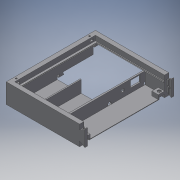
# Autodesk Inventor part: Case_side_back
Saved by Autodesk Inventor 2016 SP2 (Build 200236200, 236)
## iProperties
Created: 2018-06-26
Part Number: Case_side_back
Material: Generisch
Document SubType Name: Modeling
Designer: Nils
Density: 1 g/cm^3
Appearance: Vorgabe
Author: Nils
Autodesk Inventor part; units mm, degrees
ref_plane "YZ Plane" through (0, 0, 0) normal (1, 0, 0) x (0, 1, 0)
ref_plane "XZ Plane" through (0, 0, 0) normal (0, 1, 0) x (-1, 0, 0)
ref_plane "XY Plane" through (0, 0, 0) normal (0, 0, 1) x (1, 0, 0)
sketch "Skizze1" plane through (0, 0, 0) normal (0, 0, 1) x (1, 0, 0)
  circle A0 centre (1833.4019, 234.6963) radius 1.5 construction
  circle A1 centre (1833.4019, 396.1963) radius 1.5 construction
  line L0 (1838.4019, 230.6963) -> (1689.0019, 230.6963) construction
  line L1 (1689.0019, 230.6963) -> (1689.0019, 400.1963) construction
  line L2 (1689.0019, 400.1963) -> (1838.4019, 400.1963) construction
  line L3 (1838.4019, 400.1963) -> (1838.4019, 392.1963) construction
  line L4 (1838.4019, 392.1963) -> (1697.0019, 392.1963) construction
  line L5 (1697.0019, 392.1963) -> (1697.0019, 238.6963) construction
  line L6 (1697.0019, 238.6963) -> (1838.4019, 238.6963) construction
  line L7 (1838.4019, 238.6963) -> (1838.4019, 230.6963) construction
  line L8 (1828.4019, 390.6963) -> (1828.4019, 400.1963) construction
  line L9 (1828.4019, 230.6963) -> (1828.4019, 240.1963) construction
  line L10 (1828.4019, 230.6963) -> (1828.4019, 238.6963)
  line L11 (1828.4019, 238.6963) -> (1697.0019, 238.6963)
  line L12 (1697.0019, 238.6963) -> (1697.0019, 392.1963)
  line L13 (1828.4019, 392.1963) -> (1697.0019, 392.1963)
  line L14 (1828.4019, 392.1963) -> (1828.4019, 400.1963)
  line L15 (1828.4019, 400.1963) -> (1689.0019, 400.1963)
  line L16 (1689.0019, 400.1963) -> (1689.0019, 230.6963)
  line L17 (1689.0019, 230.6963) -> (1828.4019, 230.6963)
  circle A2 centre (1693.0019, 245.6963) radius 1.5 projected
  circle A3 centre (1693.0019, 385.1963) radius 1.5 projected
  point P0 (0, 0)
  constraints: 16 end point, 6 collinear, 4 point on line, 1 parallel
extrude "Extrusion1" add sketch "Skizze1" along normal blind 9.3 contours L17 L16 L15 L14 L13 L12 L11 L10 | A2 | A3
sketch "Skizze2" plane through (0, 0, 0) normal (0, 0, -1) x (-1, 0, 0)
  circle A0 centre (-1693.0019, 245.6963) radius 3 projected
  circle A1 centre (-1693.0019, 385.1963) radius 3 projected
  line L0 (-1689.0019, 400.1963) -> (-1689.0019, 230.6963) projected
  line L1 (-1689.0019, 230.6963) -> (-1828.4019, 230.6963) projected
  line L2 (-1828.4019, 230.6963) -> (-1828.4019, 240.1963) projected
  line L3 (-1828.4019, 240.1963) -> (-1701.0019, 240.1963) projected
  line L4 (-1701.0019, 240.1963) -> (-1701.0019, 390.6963) projected
  line L5 (-1701.0019, 390.6963) -> (-1828.4019, 390.6963) projected
  line L6 (-1828.4019, 390.6963) -> (-1828.4019, 400.1963) projected
  line L7 (-1828.4019, 400.1963) -> (-1689.0019, 400.1963) projected
  point P0 (0, 0)
extrude "Extrusion2" add sketch "Skizze2" along normal blind 2 contours A0 | A1 | L0 L1 L2 L3 L4 L5 L6 L7
chamfer "Fase1" distance 1.5 angle 45 3 edges at (1764.7019, 390.6963, -2) (1701.0019, 315.4463, -2) (1764.7019, 240.1963, -2)
sketch "Skizze3" plane through (0, 0, -2) normal (0, 0, -1) x (-1, 0, 0)
  line L0 (-1699.5019, 392.1963) -> (-1828.4019, 392.1963) projected
  line L1 (-1699.5019, 238.6963) -> (-1699.5019, 392.1963) projected
  line L2 (-1828.4019, 238.6963) -> (-1699.5019, 238.6963) projected
  line L3 (-1828.4019, 238.6963) -> (-1828.4019, 230.6963) projected
  line L4 (-1828.4019, 230.6963) -> (-1689.0019, 230.6963) projected
  line L5 (-1689.0019, 230.6963) -> (-1689.0019, 400.1963) projected
  line L6 (-1689.0019, 400.1963) -> (-1828.4019, 400.1963) projected
  line L7 (-1828.4019, 400.1963) -> (-1828.4019, 392.1963) projected
  point P0 (0, 0)
extrude "Extrusion3" add sketch "Skizze3" along normal blind 26
sketch "Skizze4" plane through (0, 0, -28) normal (0, 0, -1) x (-1, 0, 0)
  line L0 (-1828.4019, 392.1963) -> (-1828.4019, 400.1963) projected
  line L1 (-1828.4019, 392.1963) -> (-1699.5019, 392.1963)
  line L2 (-1699.5019, 392.1963) -> (-1699.5019, 238.6963)
  line L3 (-1699.5019, 238.6963) -> (-1828.4019, 238.6963)
  line L4 (-1828.4019, 238.6963) -> (-1828.4019, 392.1963)
  line L5 (-1699.5019, 392.1963) -> (-1699.5019, 238.6963) projected
  line L6 (-1699.5019, 238.6963) -> (-1828.4019, 238.6963) projected
  point P0 (0, 0)
  constraints: 8 end point, 2 collinear, 2 parallel, 1 horizontal, 1 perpendicular
extrude "Extrusion4" add sketch "Skizze4" against normal blind 3
sketch "Skizze6" plane through (0, 0, -25) normal (0, 0, 1) x (1, 0, 0)
  line L0 (1828.4019, 238.6963) -> (1697.0019, 238.6963) projected
  line L1 (1743.0019, 238.6963) -> (1745.0019, 238.6963)
  line L2 (1745.0019, 238.6963) -> (1745.0019, 317.1963)
  line L3 (1745.0019, 317.1963) -> (1743.0019, 317.1963)
  line L4 (1743.0019, 317.1963) -> (1743.0019, 238.6963)
  line L5 (1697.0019, 238.6963) -> (1697.0019, 392.1963) projected
  line L6 (1791.5019, 238.6963) -> (1791.5019, 392.1963)
  line L7 (1791.5019, 392.1963) -> (1789.0019, 392.1963)
  line L8 (1697.0019, 392.1963) -> (1828.4019, 392.1963) projected
  line L9 (1789.0019, 392.1963) -> (1789.0019, 317.1963)
  line L10 (1789.0019, 317.1963) -> (1788.5019, 317.1963)
  line L11 (1788.5019, 317.1963) -> (1788.5019, 238.6963)
  line L12 (1791.5019, 238.6963) -> (1788.5019, 238.6963)
  line L13 (1789.0019, 390.6963) -> (1789.0019, 392.1963)
  line L14 (1789.0019, 392.1963) -> (1791.5019, 392.1963)
  line L15 (1791.5019, 392.1963) -> (1791.5019, 390.6963)
  point P0 (0, 0)
  point P1 (1699.5019, 238.6963)
  dimension "d15" = 2
  dimension "d16" = 78.5
  dimension "d18" = 2.5
  dimension "d20" = 90
  dimension "d21" = 43.5
  dimension "d22" = 3
  dimension "d23" = 0.5
  dimension "d24" = 78.5
  dimension "d150" = 43.5
  constraints: 26 end point, 6 point on line, 5 perpendicular, 2 collinear, 2 parallel, 1 horizontal
  measures "d15" distance of L3.end L2.end
  measures "d16" distance of L2.end L1.end
  measures "d18" distance of L6.end L7.end
  measures "d20" angle of L9 L10
  measures "d21" distance between parallel lines of L2 L11
  measures "d22" distance between parallel lines of L11 L6
  measures "d23" distance of L9.end L10.end
  measures "d24" distance of L10.end L11.end
  measures "d150" distance of L1.start point (1699.502, 238.696)
extrude "Extrusion5" add sketch "Skizze6" along normal blind 23 contours L0 L11 L10 L9 L7 L6 | L0 L4 L3 L2
sketch "Skizze9" plane through (0, 0, -25) normal (0, 0, 1) x (1, 0, 0)
  line L0 (1828.4019, 230.6963) -> (1828.4019, 238.6963) projected
  line L1 (1828.4019, 238.6963) -> (1816.4019, 238.6963)
  line L2 (1816.4019, 238.6963) -> (1816.4019, 250.6963)
  line L3 (1816.4019, 250.6963) -> (1828.4019, 250.6963)
  line L4 (1828.4019, 250.6963) -> (1828.4019, 238.6963)
  line L5 (1828.4019, 392.1963) -> (1828.4019, 400.1963) projected
  line L6 (1828.4019, 392.1963) -> (1816.4019, 392.1963)
  line L7 (1816.4019, 392.1963) -> (1816.4019, 380.1963)
  line L8 (1816.4019, 380.1963) -> (1828.4019, 380.1963)
  line L9 (1828.4019, 380.1963) -> (1828.4019, 392.1963)
  point P0 (0, 0)
  dimension "d41" = 12
  dimension "d42" = 12
  dimension "d43" = 12
  dimension "d44" = 12
  constraints: 16 end point, 4 parallel, 2 horizontal, 2 perpendicular
  measures "d41" distance of L2.end L3.end
  measures "d42" distance of L1.end L2.end
  measures "d43" distance of L8.end L7.end
  measures "d44" distance of L7.end L6.end
extrude "Extrusion8" add sketch "Skizze9" along normal blind 8
sketch "Skizze10" plane through (0, 0, -28) normal (0, 0, -1) x (-1, 0, 0)
  line L0 (-1828.4019, 238.6963) -> (-1816.4019, 238.6963) projected
  line L1 (-1816.4019, 392.1963) -> (-1828.4019, 392.1963) projected
  line L2 (-1828.4019, 392.1963) -> (-1828.4019, 390.6963) projected
  line L3 (-1697.0019, 238.6963) -> (-1828.4019, 238.6963) projected
  line L4 (-1828.4019, 392.1963) -> (-1818.4019, 392.1963)
  line L5 (-1818.4019, 392.1963) -> (-1818.4019, 238.6963)
  line L6 (-1818.4019, 238.6963) -> (-1828.4019, 238.6963)
  line L7 (-1828.4019, 238.6963) -> (-1828.4019, 392.1963)
  point P0 (0, 0)
  dimension "d47" = 10
  constraints: 8 end point, 2 parallel, 1 horizontal, 1 perpendicular, 1 point on line
  measures "d47" distance of L5.end L6.end
extrude "Extrusion9" cut sketch "Skizze10" against normal blind 2
sketch "Skizze11" plane through (0, 0, -26) normal (0, 0, -1) x (-1, 0, 0)
  line L0 (-1828.4019, 238.6963) -> (-1828.4019, 230.6963) projected
  line L1 (-1828.4019, 238.6963) -> (-1818.4019, 238.6963)
  line L2 (-1818.4019, 238.6963) -> (-1818.4019, 248.6963)
  line L3 (-1818.4019, 248.6963) -> (-1828.4019, 248.6963)
  line L4 (-1828.4019, 248.6963) -> (-1828.4019, 238.6963)
  line L5 (-1828.4019, 392.1963) -> (-1818.4019, 392.1963) projected
  line L6 (-1828.4019, 392.1963) -> (-1818.4019, 392.1963)
  line L7 (-1818.4019, 392.1963) -> (-1818.4019, 382.1963)
  line L8 (-1818.4019, 382.1963) -> (-1828.4019, 382.1963)
  line L9 (-1828.4019, 382.1963) -> (-1828.4019, 392.1963)
  point P0 (0, 0)
  dimension "d50" = 10
  dimension "d51" = 10
  dimension "d52" = 10
  dimension "d53" = 10
  constraints: 16 end point, 4 parallel, 2 horizontal, 2 perpendicular
  measures "d50" distance of L3.end L2.end
  measures "d51" distance of L2.end L1.end
  measures "d52" distance of L7.end L8.end
  measures "d53" distance of L6.end L7.end
extrude "Extrusion10" cut sketch "Skizze11" against normal blind 3.5
sketch "Skizze12" plane through (0, 0, -22.5) normal (0, 0, -1) x (-1, 0, 0)
  line L0 (-1818.4019, 238.6963) -> (-1828.4019, 238.6963) construction
  line L1 (-1818.4019, 248.6963) -> (-1818.4019, 238.6963) construction
  line L2 (-1828.4019, 248.6963) -> (-1818.4019, 248.6963) construction
  line L3 (-1828.4019, 238.6963) -> (-1828.4019, 248.6963) construction
  line L4 (-1828.4019, 392.1963) -> (-1818.4019, 392.1963) construction
  line L5 (-1828.4019, 382.1963) -> (-1828.4019, 392.1963) construction
  line L6 (-1818.4019, 382.1963) -> (-1828.4019, 382.1963) construction
  line L7 (-1818.4019, 392.1963) -> (-1818.4019, 382.1963) construction
  circle A0 centre (-1823.4019, 243.6963) radius 1.5
  circle A1 centre (-1823.4019, 387.1963) radius 1.5
  line L8 (-1697.0019, 392.1963) -> (-1828.4019, 392.1963) construction
  line L9 (-1818.4019, 382.1963) -> (-1828.4019, 382.1963) construction
  line L10 (-1828.4019, 392.1963) -> (-1818.4019, 382.1963) construction
  line L11 (-1828.4019, 248.6963) -> (-1818.4019, 248.6963) construction
  line L12 (-1828.4019, 238.6963) -> (-1791.5019, 238.6963) construction
  line L13 (-1818.4019, 248.6963) -> (-1828.4019, 238.6963) construction
  point P0 (0, 0)
  dimension "d56" = 3
  dimension "d57" = 3
  constraints: 4 end point, 2 centre point, 2 midpoint
  measures "d56" diameter of A0
  measures "d57" diameter of A1
extrude "Extrusion11" cut sketch "Skizze12" against normal blind 9.25
sketch "Skizze13" plane through (0, 0, -17) normal (0, 0, 1) x (1, 0, 0)
  circle A0 centre (1823.4019, 243.6963) radius 1.5 projected
  circle A1 centre (1823.4019, 387.1963) radius 1.5 projected
  line L0 (1826.3019, 385.522) -> (1823.4019, 383.8476)
  line L1 (1823.4019, 383.8476) -> (1820.5019, 385.522)
  line L2 (1820.5019, 385.522) -> (1820.5019, 388.8706)
  line L3 (1820.5019, 388.8706) -> (1823.4019, 390.5449)
  line L4 (1823.4019, 390.5449) -> (1826.3019, 388.8706)
  line L5 (1826.3019, 388.8706) -> (1826.3019, 385.522)
  line L6 (1826.3019, 245.3706) -> (1826.3019, 242.022)
  line L7 (1826.3019, 242.022) -> (1823.4019, 240.3476)
  line L8 (1823.4019, 240.3476) -> (1820.5019, 242.022)
  line L9 (1820.5019, 242.022) -> (1820.5019, 245.3706)
  line L10 (1820.5019, 245.3706) -> (1823.4019, 247.0449)
  line L11 (1823.4019, 247.0449) -> (1826.3019, 245.3706)
  point P0 (0, 0)
  dimension "d64" = 5.8
  dimension "d65" = 5.8
  constraints: 24 end point, 2 coincident, 2 vertical, 26 other
  measures "d64" distance between parallel lines of L6 L9
  measures "d65" distance between parallel lines of L5 L2
extrude "Extrusion12" cut sketch "Skizze13" against normal blind 2.5
sketch "Skizze14" plane through (1689.0019, 230.6963, 9.3) normal (0, -1, 0) x (1, 0, 0)
  line L0 (139.4, 0) -> (139.4, -37.3) projected
  line L1 (139.4, -9.4235) -> (149.4, -3.65)
  line L2 (149.4, -3.65) -> (149.4, -33.65)
  line L3 (149.4, -33.65) -> (139.4, -27.8765)
  line L4 (139.4, -9.4235) -> (139.4, -27.8765)
  line L5 (139.4, 0) -> (149.4, -3.65) construction
  line L6 (149.4, -33.65) -> (139.4, -37.3) construction
  point P0 (-1689.0019, -9.3)
  dimension "d68" = 10
  dimension "d69" = 30
  dimension "d70" = 60
  dimension "d71" = 60
  constraints: 12 end point, 2 point on line, 1 collinear, 1 equal length, 1 parallel
  measures "d68" distance between parallel lines of L2 L0
  measures "d69" distance of L1.end L2.end
  measures "d70" angle of L1 L0
  measures "d71" angle of L0 L3
extrude "Extrusion13" add sketch "Skizze14" against normal blind 5
sketch "Skizze15" plane through (1689.0019, 400.1963, 9.3) normal (0, 1, 0) x (1, 0, 0)
  line L0 (139.4, 9.4235) -> (139.4, 27.8765) projected
  line L1 (139.4, 9.4235) -> (149.4, 3.65) projected
  line L2 (149.4, 3.65) -> (149.4, 33.65) projected
  line L3 (149.4, 33.65) -> (139.4, 27.8765) projected
  point P0 (-1689.0019, 9.3)
extrude "Extrusion14" add sketch "Skizze15" against normal blind 5
sketch "Skizze16" plane through (1789.0019, 317.1963, -28) normal (-1, 0, 0) x (0, 0, 1)
  line L0 (12, 30) -> (17, 30)
  line L1 (17, 30) -> (17, 35)
  line L2 (17, 35) -> (12, 35)
  line L3 (12, 35) -> (12, 30)
  line L4 (3, 0) -> (26, 0) projected
  line L5 (26, 75) -> (26, 0) projected
  point P0 (28, -317.1963)
  dimension "d76" = 5
  dimension "d77" = 5
  dimension "d217" = 30
  dimension "d218" = 9
  constraints: 8 end point, 2 parallel, 1 horizontal, 1 perpendicular
  measures "d76" distance of L2.end L1.end
  measures "d77" distance of L1.end L0.end
  measures "d217" distance between parallel lines of L4 L0
  measures "d218" distance between parallel lines of L5 L1
extrude "Extrusion15" cut sketch "Skizze16" against normal blind 2.5
sketch "Skizze17" plane through (1689.0019, 230.6963, 9.3) normal (-1, 0, 0) x (0, 0, 1)
  line L0 (-33.65, 0) -> (-3.65, 0) construction
  line L1 (-18.65, 0) -> (-18.65, 86.5) construction
  line L2 (-34.3, 86.5) -> (-11.3, 86.5) construction
  circle A0 centre (-18.65, 76.5) radius 5
  circle A1 centre (-18.65, 51.5) radius 5
  point P0 (-9.3, -230.6963)
  dimension "d82" = 10
  dimension "d83" = 10
  dimension "d84" = 25
  dimension "d85" = 10
  constraints: 3 point on line, 2 centre point, 2 end point, 1 midpoint, 1 vertical
  measures "d82" diameter of A0
  measures "d83" diameter of A1
  measures "d84" distance of A1.centre A0.centre
  measures "d85" distance from line of L2 A0.centre
extrude "Extrusion16" cut sketch "Skizze17" against normal blind 4
sketch "Skizze18" plane through (0, 0, 9.3) normal (0, 0, 1) x (1, 0, 0)
  circle A0 centre (1693.0019, 245.6963) radius 1.5 projected
  circle A1 centre (1693.0019, 385.1963) radius 1.5 projected
  point P0 (0, 0)
extrude "Extrusion17" cut sketch "Skizze18" against normal blind 9
sketch "Skizze19" plane through (1697.0019, 238.6963, 9.3) normal (1, 0, 0) x (0, 0, -1)
  line L0 (0, 8.5) -> (9, 8.5) construction
  line L1 (0, 5.5) -> (9, 5.5) construction
  line L2 (0, 148) -> (9, 148) construction
  line L3 (0, 145) -> (9, 145) construction
  line L4 (3.5, 143.65) -> (6.5, 143.65)
  line L5 (6.5, 143.65) -> (6.5, 149.35)
  line L6 (6.5, 149.35) -> (3.5, 149.35)
  line L7 (3.5, 149.35) -> (3.5, 143.65)
  line L8 (3.5, 9.85) -> (6.5, 9.85)
  line L9 (6.5, 9.85) -> (6.5, 4.15)
  line L10 (6.5, 4.15) -> (3.5, 4.15)
  line L11 (3.5, 4.15) -> (3.5, 9.85)
  line L12 (5, 4.15) -> (5, 5.5) construction
  line L13 (5, 8.5) -> (5, 9.85) construction
  line L14 (0, 0) -> (0, 153.5) construction
  point P0 (9.3, -238.6963)
  dimension "d90" = 3
  dimension "d91" = 5.7
  dimension "d92" = 3
  dimension "d93" = 5.7
  dimension "d94" = 1.35
  dimension "d95" = 3.5
  dimension "d98" = 1.35
  constraints: 20 end point, 4 parallel, 4 point on line, 3 perpendicular, 2 horizontal, 2 midpoint, 1 collinear
  measures "d90" distance of L6.end L5.end
  measures "d91" distance of L5.end L4.end
  measures "d92" distance of L9.end L10.end
  measures "d93" distance of L8.end L9.end
  measures "d94" distance between parallel lines of L6 L2
  measures "d95" distance between parallel lines of L7 L14
  measures "d98" distance between parallel lines of L8 L0
extrude "Extrusion18" cut sketch "Skizze19" against normal blind 7
sketch "Skizze20" plane through (0, 0, 9.3) normal (0, 0, 1) x (1, 0, 0)
  circle A0 centre (1833.4019, 234.6963) radius 1.5 projected
  circle A1 centre (1833.4019, 396.1963) radius 1.5 projected
  point P0 (0, 0)
extrude "Extrusion19" cut sketch "Skizze20" against normal blind 62.25
sketch "Skizze21" plane through (1689.0019, 235.6963, 9.3) normal (0, 1, 0) x (1, 0, 0)
  line L0 (139.4, 9.4235) -> (139.4, 27.8765) construction
  line L1 (139.4, 18.65) -> (149.4, 18.65) construction
  line L2 (149.4, 3.65) -> (149.4, 33.65) construction
  line L3 (141.55, 17.25) -> (147.25, 17.25)
  line L4 (147.25, 17.25) -> (147.25, 20.05)
  line L5 (147.25, 20.05) -> (141.55, 20.05)
  line L6 (141.55, 20.05) -> (141.55, 17.25)
  line L7 (141.55, 17.25) -> (147.25, 20.05) construction
  line L8 (147.25, 17.25) -> (141.55, 20.05) construction
  point P0 (144.4, 18.65)
  dimension "d101" = 5.7
  dimension "d102" = 2.8
  constraints: 14 end point, 5 midpoint, 2 parallel, 1 horizontal, 1 perpendicular
  measures "d101" distance of L5.end L4.end
  measures "d102" distance of L4.end L3.end
extrude "Extrusion20" cut sketch "Skizze21" against normal blind 4
sketch "Skizze22" plane through (1689.0019, 395.1963, 9.3) normal (0, -1, 0) x (1, 0, 0)
  line L0 (147.25, -17.25) -> (141.55, -17.25) projected
  line L1 (147.25, -20.05) -> (147.25, -17.25) projected
  line L2 (141.55, -20.05) -> (147.25, -20.05) projected
  line L3 (141.55, -17.25) -> (141.55, -20.05) projected
  point P0 (-1689.0019, -9.3)
extrude "Extrusion21" cut sketch "Skizze22" against normal blind 4
sketch "Skizze27" plane through (1689.0019, 230.6963, 9.3) normal (-1, 0, 0) x (0, 0, 1)
  line L0 (-11.3, 161.5) -> (-11.3, 86.5) construction
  line L1 (-37.3, 161.5) -> (-37.3, 8) projected
  line L2 (-37.3, 86.5) -> (-27.3, 86.5)
  line L3 (-27.3, 86.5) -> (-27.3, 154.5)
  line L4 (-27.3, 154.5) -> (-11.3, 154.5)
  line L5 (-11.3, 154.5) -> (-11.3, 169.5)
  line L6 (-11.3, 169.5) -> (-37.3, 169.5)
  line L7 (-37.3, 169.5) -> (-37.3, 86.5)
  line L8 (0, 169.5) -> (-37.3, 169.5) projected
  line L9 (-34.3, 86.5) -> (-11.3, 86.5) construction
  point P0 (-9.3, -230.6963)
  dimension "d151" = 10
  dimension "d152" = 15
  constraints: 12 end point, 3 collinear, 3 perpendicular, 2 point on line, 1 vertical
  measures "d151" distance of L2.start L2.end
  measures "d152" distance between parallel lines of L6 L4
extrude "Extrusion22" cut sketch "Skizze27" against normal blind 100
sketch "Skizze28" plane through (1699.5019, 238.6963, -2) normal (1, 0, 0) x (0, 0, -1)
  line L0 (16, 78.5) -> (16, 146.5) projected
  line L1 (16, 82.8199) -> (21, 81)
  line L2 (21, 81) -> (21, 91)
  line L3 (21, 91) -> (16, 89.1801)
  line L4 (0, 146.5) -> (0, 153.5) projected
  line L5 (5, 159) -> (0, 157.1801)
  line L6 (0, 161.5) -> (0, 146.5) projected
  line L7 (0, 150.8199) -> (5, 149)
  line L8 (5, 149) -> (5, 159)
  line L9 (23, 78.5) -> (16, 78.5) projected
  point P0 (-2, -238.6963)
  dimension "d156" = 5
  dimension "d157" = 70
  dimension "d158" = 70
  dimension "d159" = 10
  dimension "d162" = 70
  dimension "d163" = 10
  dimension "d164" = 70
  dimension "d165" = 2.5
  dimension "d166" = 5
  dimension "d167" = 2.5
  constraints: 12 end point, 4 point on line, 2 parallel, 1 vertical
  measures "d156" distance between parallel lines of L0 L2
  measures "d157" angle of L3 L0
  measures "d158" angle of L0 L1
  measures "d159" distance of L1.end L2.end
  measures "d162" angle of L5 L6
  measures "d163" distance of L7.end L5.start
  measures "d164" angle of L7 L4
  measures "d165" vertical distance of L6.start L5.start
  measures "d166" distance between parallel lines of L8 L6
  measures "d167" distance from line of L1.end L9
extrude "Extrusion23" add sketch "Skizze28" against normal blind 6
sketch "Skizze29" plane through (1789.0019, 317.1963, -28) normal (-1, 0, 0) x (0, 0, 1)
  line L0 (5, 12.5) -> (5, 2.5) construction
  line L1 (5, 7.5) -> (5, 7.5) construction
  line L2 (21, 70.5) -> (21, 80.5) construction
  line L3 (21, 75.5) -> (0, 75.5) construction
  circle A0 centre (5, 75.5) radius 3.5
  circle A1 centre (5, 7.5) radius 3.5
  line L4 (0, 83) -> (26, 83) projected
  line L5 (0, 0) -> (0, 83) projected
  dimension "d170" = 7
  dimension "d171" = 7
  dimension "d172" = 7.5
  dimension "d173" = 5
  dimension "d174" = 5
  constraints: 4 end point, 3 midpoint, 2 centre point, 2 horizontal, 1 point on line
  measures "d170" diameter of A0
  measures "d171" diameter of A1
  measures "d172" distance from line of L4 A0.centre
  measures "d173" distance from line of L5 A0.centre
  measures "d174" distance from line of L5 A1.centre
extrude "Extrusion24" cut sketch "Skizze29" against normal blind 2.5
thread "Gewinde3" size "M10x1.5" class "6H" standard "ANSI Metric M Profile" full length
thread "Gewinde4" size "M10x1.5" class "6H" standard "ANSI Metric M Profile" full length
sketch "Skizze31" plane through (1693.0019, 307.1963, -9.35) normal (0, -1, 0) x (0, 0, 1)
  line L0 (5, 0) -> (5, 4)
  line L1 (5, 4) -> (4.0211, 4)
  line L2 (4.0211, 4) -> (4.0211, 0)
  line L3 (4.0211, 0) -> (5, 0)
  line L4 (0, -0.8) -> (0, 4.8) projected
  constraints: 8 end point
revolve "Umdrehung3" add sketch "Skizze31" angle 360 about axis through (1693.0019, 307.1963, -9.35) along (-1, 0, 0) separate body
sketch "Skizze30" plane through (1693.0019, 307.1963, -4.35) normal (0, 1, 0) x (-1, 0, 0)
  line L0 (-0.8887, -0.0802) -> (-0.7501, -0.0802) construction
  line L1 (0.1385, -0.899) -> (-0.0001, -1.1391) construction
  line L2 (-1.5001, -1.1391) -> (-1.6387, -0.899) construction
  line L3 (-0.6115, -0.0802) -> (-0.7501, 0.1599) construction
  line L4 (-0.7501, 0.1599) -> (-0.8887, -0.0802) construction
  line L5 (-1.5001, -1.1391) -> (-1.3615, -0.899) construction
  line L6 (-0.6115, -0.0802) -> (-0.1387, -0.899)
  line L7 (-1.6387, -0.899) -> (-1.3615, -0.899) construction
  arc A0 (-1.6387, -0.899) -> (-1.5001, -0.979) centre (-1.5001, -0.819) ccw construction
  line L8 (0.1385, -0.899) -> (-0.1387, -0.899) construction
  line L9 (-1.5001, -1.1391) -> (-1.5001, -0.899) construction
  line L10 (-0.0001, -1.1391) -> (-0.0001, -0.899) construction
  line L11 (-0.7501, 0.1599) -> (-0.7501, -0.0002) construction
  line L12 (-1.5001, -0.979) -> (-0.0001, -0.979)
  arc A1 (-1.5001, -0.979) -> (-1.3615, -0.899) centre (-1.5001, -0.819) ccw
  line L13 (-0.1387, -0.899) -> (-0.0001, -1.1391) construction
  line L14 (-1.3615, -0.899) -> (-0.8887, -0.0802)
  line L15 (-0.0001, -0.0002) -> (-0.0001, 0.0177)
  line L16 (-0.0001, 0.0177) -> (-0.0001, -0.0002)
  line L17 (-0.0001, -0.0002) -> (0.0334, -0.0002)
  arc A2 (-0.1387, -0.899) -> (-0.0001, -0.979) centre (-0.0001, -0.819) ccw
  arc A3 (-0.0001, -0.979) -> (0.1385, -0.899) centre (-0.0001, -0.819) ccw construction
  arc A4 (-0.7501, -0.0002) -> (-0.8887, -0.0802) centre (-0.7501, -0.1603) ccw
  arc A5 (-0.6115, -0.0802) -> (-0.7501, -0.0002) centre (-0.7501, -0.1603) ccw
  line L18 (-0.7501, -0.0002) -> (-0.7501, -0.0802) construction
  line L19 (-0.7501, -0.0802) -> (-0.6115, -0.0802) construction
  dimension "d181" = 60
  dimension "d182" = 0.2401
  dimension "d183" = 0.2401
  dimension "Skizze30_ThreadOffset" = 0
  dimension "Skizze30_MajorRadius" = 0.9789
  dimension "d186" = 1.5
  dimension "Skizze30_MinorRadius" = 0
  constraints: 40 end point, 12 point on circle, 10 parallel, 8 tangent, 6 centre point, 6 collinear, 2 midpoint, 2 point on line, 1 horizontal, 1 perpendicular, 3 other
  measures "d181" angle of L6 L14
  measures "d182" distance of L3.end L0.end
  measures "d183" distance of L1.end L10.end
  measures "Skizze30_ThreadOffset" distance between parallel lines of L15 L10
  measures "Skizze30_MajorRadius" distance from line of L12 L15.start
  measures "d186" distance from line of L1.end L9
  measures "Skizze30_MinorRadius" distance edge to line of A5 L17
coil "Spirale3" sketch "Skizze30" operation cut axis through (1693.0019, 307.1963, -9.35) along (-1, 0, 0) pitch 1.5015 turns 4.662005 hand right bodies 2
sketch "Skizze33" plane through (1693.0019, 282.1963, -9.35) normal (0, -1, 0) x (0, 0, 1)
  line L0 (5, 0) -> (5, 4)
  line L1 (5, 4) -> (4.0211, 4)
  line L2 (4.0211, 4) -> (4.0211, 0)
  line L3 (4.0211, 0) -> (5, 0)
  line L4 (0, -0.8) -> (0, 4.8) projected
  constraints: 8 end point
revolve "Umdrehung4" add sketch "Skizze33" angle 360 about axis through (1693.0019, 282.1963, -9.35) along (-1, 0, 0) separate body
sketch "Skizze32" plane through (1693.0019, 282.1963, -4.35) normal (0, 1, 0) x (-1, 0, 0)
  line L0 (-0.8887, -0.0802) -> (-0.7501, -0.0802) construction
  line L1 (0.1385, -0.899) -> (-0.0001, -1.1391) construction
  line L2 (-1.5001, -1.1391) -> (-1.6387, -0.899) construction
  line L3 (-0.6115, -0.0802) -> (-0.7501, 0.1599) construction
  line L4 (-0.7501, 0.1599) -> (-0.8887, -0.0802) construction
  line L5 (-1.5001, -1.1391) -> (-1.3615, -0.899) construction
  line L6 (-0.6115, -0.0802) -> (-0.1387, -0.899)
  line L7 (-1.6387, -0.899) -> (-1.3615, -0.899) construction
  arc A0 (-1.6387, -0.899) -> (-1.5001, -0.979) centre (-1.5001, -0.819) ccw construction
  line L8 (0.1385, -0.899) -> (-0.1387, -0.899) construction
  line L9 (-1.5001, -1.1391) -> (-1.5001, -0.899) construction
  line L10 (-0.0001, -1.1391) -> (-0.0001, -0.899) construction
  line L11 (-0.7501, 0.1599) -> (-0.7501, -0.0002) construction
  line L12 (-1.5001, -0.979) -> (-0.0001, -0.979)
  arc A1 (-1.5001, -0.979) -> (-1.3615, -0.899) centre (-1.5001, -0.819) ccw
  line L13 (-0.1387, -0.899) -> (-0.0001, -1.1391) construction
  line L14 (-1.3615, -0.899) -> (-0.8887, -0.0802)
  line L15 (-0.0001, -0.0002) -> (-0.0001, 0.0177)
  line L16 (-0.0001, 0.0177) -> (-0.0001, -0.0002)
  line L17 (-0.0001, -0.0002) -> (0.0334, -0.0002)
  arc A2 (-0.1387, -0.899) -> (-0.0001, -0.979) centre (-0.0001, -0.819) ccw
  arc A3 (-0.0001, -0.979) -> (0.1385, -0.899) centre (-0.0001, -0.819) ccw construction
  arc A4 (-0.7501, -0.0002) -> (-0.8887, -0.0802) centre (-0.7501, -0.1603) ccw
  arc A5 (-0.6115, -0.0802) -> (-0.7501, -0.0002) centre (-0.7501, -0.1603) ccw
  line L18 (-0.7501, -0.0002) -> (-0.7501, -0.0802) construction
  line L19 (-0.7501, -0.0802) -> (-0.6115, -0.0802) construction
  dimension "d199" = 60
  dimension "d200" = 0.2401
  dimension "d201" = 0.2401
  dimension "Skizze32_ThreadOffset" = 0
  dimension "Skizze32_MajorRadius" = 0.9789
  dimension "d204" = 1.5
  dimension "Skizze32_MinorRadius" = 0
  constraints: 40 end point, 12 point on circle, 10 parallel, 8 tangent, 6 centre point, 6 collinear, 2 midpoint, 2 point on line, 1 horizontal, 1 perpendicular, 3 other
  measures "d199" angle of L6 L14
  measures "d200" distance of L3.end L0.end
  measures "d201" distance of L1.end L10.end
  measures "Skizze32_ThreadOffset" distance between parallel lines of L15 L10
  measures "Skizze32_MajorRadius" distance from line of L12 L15.start
  measures "d204" distance from line of L1.end L9
  measures "Skizze32_MinorRadius" distance edge to line of A5 L17
coil "Spirale4" sketch "Skizze32" operation cut axis through (1693.0019, 282.1963, -9.35) along (-1, 0, 0) pitch 1.5015 turns 4.662005 hand right bodies 3
sketch "Skizze34" plane through (1789.0019, 317.1963, -28) normal (-1, 0, 0) x (0, 0, 1)
  line L0 (11.5, 47) -> (24, 47)
  line L1 (24, 47) -> (24, 66)
  line L2 (24, 66) -> (11.5, 66)
  line L3 (11.5, 66) -> (11.5, 47)
  line L4 (12, 35) -> (17, 35) projected
  line L5 (26, 75) -> (26, 0) projected
  circle A0 centre (5, 75.5) radius 3.5 projected
  line L6 (17.75, 66) -> (17.75, 47) construction
  line L7 (10.25, 46.25) -> (25.25, 46.25) construction
  line L8 (25.25, 46.25) -> (25.25, 66.75) construction
  line L9 (25.25, 66.75) -> (10.25, 66.75) construction
  line L10 (10.25, 66.75) -> (10.25, 46.25) construction
  line L11 (10.25, 46.25) -> (25.25, 66.75) construction
  line L12 (25.25, 46.25) -> (10.25, 66.75) construction
  line L13 (9, 0.1) -> (9, 74) construction
  line L14 (9, 74) -> (25.8, 74) construction
  point P0 (28, -317.1963)
  point P1 (17.75, 56.5)
  dimension "d219" = 12.5
  dimension "d220" = 19
  dimension "d221" = 12
  dimension "d222" = 2
  dimension "d223" = 6.5
  dimension "d231" = 15
  dimension "d232" = 20.5
  constraints: 22 end point, 5 midpoint, 4 parallel, 2 horizontal, 2 perpendicular
  measures "d219" distance of L2.end L1.end
  measures "d220" distance of L1.end L0.end
  measures "d221" distance between parallel lines of L4 L0
  measures "d222" distance between parallel lines of L5 L1
  measures "d223" distance from line of A0.centre L3
  measures "d231" distance of L9.end L8.end
  measures "d232" distance of L8.end L7.end
extrude "Extrusion25" cut sketch "Skizze34" against normal blind 10 contours L3 L2 L1 L0 bodies 1
sketch "Skizze35" plane through (0, 0, -2) normal (0, 0, 1) x (1, 0, 0)
  line L0 (1697.0019, 238.6963) -> (1828.4019, 238.6963) projected
  line L1 (1828.4019, 238.6963) -> (1828.4019, 240.1963) projected
  line L2 (1828.4019, 240.1963) -> (1701.0019, 240.1963) projected
  line L3 (1701.0019, 240.1963) -> (1701.0019, 390.6963) projected
  line L4 (1701.0019, 390.6963) -> (1828.4019, 390.6963) projected
  line L5 (1828.4019, 390.6963) -> (1828.4019, 392.1963) projected
  line L6 (1828.4019, 392.1963) -> (1697.0019, 392.1963) projected
  line L7 (1697.0019, 392.1963) -> (1697.0019, 238.6963) projected
  point P0 (0, 0)
extrude "Extrusion26" add sketch "Skizze35" along normal blind 0.75 bodies 1
chamfer "Fase2" distance 0.75 angle 45 3 edges at (1764.7019, 240.1963, -1.25) (1701.0019, 315.4463, -1.25) (1764.7019, 390.6963, -1.25)
equation "\"d21\" = d17"
equation "\"d42\" = d41"
equation "\"d43\" = d41"
equation "\"d44\" = d41"
equation "\"d51\" = d50"
equation "\"d52\" = d50"
equation "\"d53\" = d50"
equation "\"d56\" = d57"
equation "\"d83\" = d82"
equation "\"d90\" = d92"
equation "\"d91\" = d93"
equation "\"d94\" = d98"
equation "\"d157\" = d164"
equation "\"d158\" = d157"
equation "\"d170\" = d171"
equation "\"d174\" = d173"
equation "\"d181\" = d188"
equation "\"d182\" = 0.160083 * Skizze30_Pitch"
equation "\"d183\" = 0.160083 * Skizze30_Pitch"
equation "\"d186\" = Skizze30_Pitch"
equation "\"d199\" = d206"
equation "\"d200\" = 0.160083 * Skizze32_Pitch"
equation "\"d201\" = 0.160083 * Skizze32_Pitch"
equation "\"d204\" = Skizze32_Pitch"
equation "\"d118\" = 60deg"
equation "\"Skizze23_Pitch\" = 1.5"
equation "\"d136\" = 60deg"
equation "\"Skizze25_Pitch\" = 1.5"
equation "\"d188\" = 60deg"
equation "\"Skizze30_Pitch\" = 1.5"
equation "\"d206\" = 60deg"
equation "\"Skizze32_Pitch\" = 1.5"
equation "\"d17\" = 43.5"
